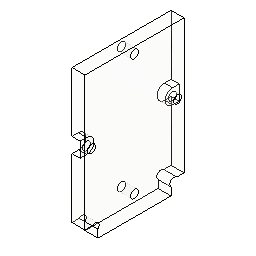
AssemblyThrowerNew v12 (Autodesk Fusion 360 archive; units mm, degrees)
design "RampBack"
Autodesk Fusion 360 part; units mm, degrees
sketch "Sketch1" plane through (0, 0, 0) normal (1, 0, 0) x (0, 1, 0)
  line L0 (-18.3, 27.3) -> (18.3, 27.3)
  line L1 (18.3, 27.3) -> (18.3, -22.3)
  line L2 (13.5, -27.3) -> (-13.5, -27.3)
  line L3 (-18.3, -22.3) -> (-18.3, 27.3)
  line L4 (0, 0) -> (0, 27.3) construction
  line L5 (-13.5, 27.3) -> (-13.5, -22.3) construction
  line L6 (13.5, 27.3) -> (13.5, -22.3) construction
  line L7 (-18.3, 22.5) -> (18.3, 22.5) construction
  line L8 (-18.3, -17.5) -> (18.3, -17.5) construction
  line L9 (-13.5, -22.3) -> (13.5, -22.3) construction
  line L10 (-18.3, 2.5) -> (18.3, 2.5) construction
  line L11 (0, 0) -> (0, -19.9) construction
  circle A0 centre (0, -19.9) radius 1.5
  circle A1 centre (-15.9, 2.5) radius 1.5
  circle A2 centre (15.9, 2.5) radius 1.5
  circle A3 centre (0, 24.9) radius 1.5
  line L12 (-18.3, -22.3) -> (-15.6213, -22.3)
  line L13 (-13.5, -24.4213) -> (-13.5, -27.3)
  line L14 (13.5, -24.4213) -> (13.5, -27.3)
  line L15 (15.6213, -22.3) -> (18.3, -22.3)
  line L16 (-18.3, -27.3) -> (-18.3, -22.3) construction
  line L17 (-13.5, -27.3) -> (-18.3, -27.3) construction
  line L18 (18.3, -27.3) -> (13.5, -27.3) construction
  line L19 (0, 0) -> (18.3, 0)
  line L20 (18.3, -22.3) -> (18.3, -27.3) construction
  line L21 (-13.5, -22.3) -> (-14.5607, -23.3607) construction
  arc A4 (-13.5, -24.4213) -> (-15.6213, -22.3) centre (-14.5607, -23.3607) ccw
  arc A5 (-15.6213, -22.3) -> (-13.5, -24.4213) centre (-14.5607, -23.3607) ccw construction
  line L22 (-13.5, -22.3) -> (-13.5, -24.4213) construction
  line L23 (-15.6213, -22.3) -> (-13.5, -22.3) construction
  line L24 (13.5, -22.3) -> (14.5607, -23.3607) construction
  arc A6 (15.6213, -22.3) -> (13.5, -24.4213) centre (14.5607, -23.3607) ccw
  arc A7 (13.5, -24.4213) -> (15.6213, -22.3) centre (14.5607, -23.3607) ccw construction
  line L25 (13.5, -22.3) -> (15.6213, -22.3) construction
  line L26 (13.5, -22.3) -> (13.5, -24.4213) construction
  line L27 (-15.9, -0.25) -> (-18.3, -0.25)
  line L28 (-15.9, 5.25) -> (-18.3, 5.25)
  arc A8 (-15.9, -0.25) -> (-15.9, 5.25) centre (-15.9, 2.5) ccw
  arc A9 (-15.9, 5.25) -> (-18.3, 3.8426) centre (-15.9, 2.5) ccw construction
  arc A10 (-18.3, 3.8426) -> (-18.3, 1.1574) centre (-15.9, 2.5) ccw construction
  arc A11 (-18.3, 1.1574) -> (-15.9, -0.25) centre (-15.9, 2.5) ccw construction
  line L29 (15.9, 5.25) -> (18.3, 5.25)
  line L30 (15.9, -0.25) -> (18.3, -0.25)
  arc A12 (15.9, -0.25) -> (15.9, 5.25) centre (15.9, 2.5) ccw construction
  arc A13 (14.7544, 0) -> (15.9, -0.25) centre (15.9, 2.5) ccw
  arc A14 (13.5, 1.1574) -> (14.7544, 0) centre (15.9, 2.5) ccw
  arc A15 (13.15, 2.5) -> (13.5, 1.1574) centre (15.9, 2.5) ccw
  arc A16 (13.5, 3.8426) -> (13.15, 2.5) centre (15.9, 2.5) ccw
  arc A17 (15.9, 5.25) -> (13.5, 3.8426) centre (15.9, 2.5) ccw
  point P0 (18.3, 0)
  dimension "d20" = 4.8
  dimension "d21" = 4.8
  dimension "d22" = 4.8
  dimension "d23" = 27
  dimension "d24" = 4.8
  dimension "d25" = 5
  dimension "d26" = 40
  dimension "d27" = 20
  dimension "d28" = 2.4
  dimension "d29" = 3
  dimension "d30" = 3
  dimension "d31" = 3
  dimension "d32" = 3
  dimension "d33" = 2.4
  dimension "d34" = 2.4
  dimension "d35" = 2.4
  dimension "d38" = 2.5
  dimension "d39" = 1.5
  dimension "d40" = 45
  dimension "d41" = 3
  dimension "d42" = 1.5
  dimension "d43" = 45
  dimension "d44" = 3
  dimension "d45" = 5.5
  dimension "d46" = 5.5
  constraint horizontal L0
  constraint vertical L1
  constraint horizontal L2
  constraint vertical L3
  constraint coincident L4.start L11.start
  constraint midpoint L0 L4.end
  constraint vertical L4
  constraint coincident L0 L5.start
  constraint perpendicular L2 L5
  constraint coincident L0 L6.start
  constraint perpendicular L2 L6
  constraint coincident L3 L7.start
  constraint coincident L1 L7.end
  constraint perpendicular L1 L7
  constraint coincident L3 L8.start
  constraint coincident L1 L8.end
  constraint perpendicular L1 L8
  constraint perpendicular L1 L9
  constraint coincident L3 L10.start
  constraint coincident L1 L10.end
  constraint perpendicular L1 L10
  constraint perpendicular L8 L11
  constraint coincident L11.end A0.centre
  constraint coincident L10 A1.centre
  constraint coincident L10 A2.centre
  constraint coincident L4 A3.centre
  constraint perpendicular L1 L12
  constraint perpendicular L2 L13
  constraint perpendicular L2 L14
  constraint perpendicular L1 L15
  constraint vertical L16
  constraint horizontal L17
  constraint horizontal L18
  constraint coincident L1 P0
  constraint coincident P0 L19.end
  constraint perpendicular L1 L19
  constraint vertical L20
  constraint coincident L21.end A4.centre
  constraint concentric A4 A5
  constraint perpendicular L2 L22
  constraint perpendicular L1 L23
  constraint coincident L24.end A6.centre
  constraint concentric A6 A7
  constraint perpendicular L1 L25
  constraint perpendicular L2 L26
  constraint concentric A1 A8
  constraint coincident L3 L27.end
  constraint tangent L27 A8
  constraint horizontal L27
  constraint coincident L3 L28.end
  constraint perpendicular L3 L28
  constraint tangent L28 A8
  constraint coincident L3 A9.end
  constraint concentric A8 A9
  constraint coincident L3 A10.end
  constraint concentric A8 A10
  constraint concentric A8 A11
  constraint concentric A2 A12
  constraint coincident L1 L29.end
  constraint perpendicular L1 L29
  constraint tangent L29 A12
  constraint coincident L1 L30.end
  constraint horizontal L30
  constraint tangent L30 A12
  constraint coincident L19 A13.start
  constraint concentric A12 A13
  constraint coincident L6 A14.start
  constraint concentric A12 A14
  constraint coincident L10 A15.start
  constraint concentric A12 A15
  constraint coincident L6 A16.start
  constraint concentric A12 A16
  constraint concentric A12 A17
  measures "d20" distance of L3 L5
  measures "d21" distance of L1 L6
  measures "d22" distance of L0 L7
  measures "d23" distance of L5 L6
  measures "d24" distance of L8 L9
  measures "d25" distance of L2 L9
  measures "d26" distance of L7 L8
  measures "d27" distance of L7 L10
  measures "d28" distance of L8 L11.end
  measures "d29" diameter of A0
  measures "d30" diameter of A1
  measures "d31" diameter of A2
  measures "d32" diameter of A3
  measures "d33" distance of L0 A3.centre
  measures "d34" distance of L3 A1.centre
  measures "d35" distance of L1 A2.centre
  measures "d38" distance of L10 P0
  measures "d39" distance of L5.end L21.end
  measures "d40" angle of L12 L21
  measures "d41" diameter of A4
  measures "d42" distance of L6.end L24.end
  measures "d43" angle of L15 L24
  measures "d44" diameter of A6
  measures "d45" diameter of A8
  measures "d46" diameter of A12
extrude "Extrude1" add sketch "Sketch1" along normal blind 4.8
extrude "Extrude2" cut sketch "Sketch1" along normal blind 3 contours L3 L27 L28 A8 | L1 L19 L29 A14 A15 A16 A17 | L1 L19 L30 A13

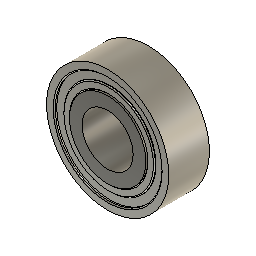
design "RollerBearing12x5x4"
Autodesk Fusion 360 part; units mm, degrees
sketch "Sketch1" plane through (0, 0, 0) normal (0, 1, 0) x (1, 0, 0)
  circle A0 centre (0, 0) radius 2.5
  circle A1 centre (0, 0) radius 3.75
  circle A2 centre (0, 0) radius 6
  circle A3 centre (0, 0) radius 5.25
  circle A4 centre (0, 0) radius 4.5
  dimension "d1" = 5
  dimension "d2" = 7.5
  dimension "d3" = 12
  dimension "d4" = 10.5
  dimension "d13" = 9
  constraint coincident A0.centre A1.centre
  constraint concentric A1 A2
  constraint concentric A1 A3
  constraint concentric A2 A4
  measures "d1" diameter of A0
  measures "d2" diameter of A1
  measures "d3" diameter of A2
  measures "d4" diameter of A3
  measures "d13" diameter of A4
extrude "Extrude1" add sketch "Sketch1" along normal blind 4 contours A2 | A3 | A4 makes body 1
extrude "Extrude2" add sketch "Sketch1" along normal blind 4 separate body contours A1 makes body 2
extrude "Extrude3" cut sketch "Sketch1" along normal blind 0.25 contours A3 bodies 1
sketch "Sketch2" plane through (0, 4, 0) normal (0, 1, 0) x (-1, 0, 0)
  circle A0 centre (0, 0) radius 3.75
  circle A1 centre (0, 0) radius 6
  circle A2 centre (0, 0) radius 5.25
  circle A3 centre (0, 0) radius 4.5
extrude "Extrude4" cut sketch "Sketch2" against normal blind 0.25 contours A2 bodies 1
extrude "Extrude5" cut 1 faces at (4.2193, 0, 0.4099) along direction (0, 1, 0) blind 0.1 on bodies 1 bodies 1
extrude "Extrude6" cut 1 faces at (-4.2193, 4, -0.4099) along direction (0, -1, 0) blind 0.1 on bodies 1 bodies 1
fillet "Fillet2" radius 0.1 6 edges at (-3.4962, 3.9, 1.3561) (4.1955, 3.9, 1.6273) (4.8947, 4, 1.8985) (-4.8947, 0, 1.8985) (-4.1955, 0.1, 1.6273) (-3.4962, 0.1, -1.3561) on bodies 1

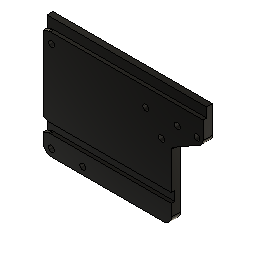
design "ThrowerStatorSidePlate"
Autodesk Fusion 360 part; units mm, degrees
sketch "Sketch1" plane through (0, 0, 0) normal (0, 1, 0) x (1, 0, 0)
  circle A0 centre (0, 0) radius 48 construction
  circle A1 centre (0, 0) radius 14 construction
  circle A2 centre (0, 0) radius 9.5 construction
  circle A3 centre (0, 0) radius 8 construction
  line L0 (0, 0) -> (8, 0) construction
  line L1 (0, 0) -> (0, -9.5) construction
  line L2 (0, 0) -> (-8, 0) construction
  line L3 (0, 0) -> (0, 9.5) construction
  circle A4 centre (8, 0) radius 1.5
  circle A5 centre (-8, 0) radius 1.5
  circle A6 centre (0, 9.5) radius 1.5
  circle A7 centre (0, 0) radius 12 construction
  line L4 (8, 0) -> (18, 0) construction
  line L5 (21.1, 0) -> (19.55, 2.6847) construction
  line L6 (19.55, 2.6847) -> (16.45, 2.6847) construction
  line L7 (16.45, 2.6847) -> (14.9, 0) construction
  line L8 (14.9, 0) -> (16.45, -2.6847) construction
  line L9 (16.45, -2.6847) -> (19.55, -2.6847) construction
  line L10 (19.55, -2.6847) -> (21.1, 0) construction
  circle A8 centre (18, 0) radius 3.1 construction
  circle A9 centre (18, 0) radius 1.5
  line L11 (0, 52) -> (-68, 52) construction
  line L12 (-9.7468, 47) -> (-68, 47) construction
  line L13 (-68, 52) -> (-68, 47) construction
  line L14 (-68, 47) -> (-68, 35.633) construction
  line L15 (-68, 35.633) -> (-32.1604, 35.633) construction
  line L16 (-68, 35.633) -> (-68, 30.833) construction
  line L17 (-68, 30.833) -> (-36.7876, 30.833) construction
  line L18 (-68, 30.833) -> (-68, -9.167) construction
  line L19 (-60, -9.167) -> (-47.1165, -9.167)
  line L20 (-68, -9.167) -> (-68, -13.967) construction
  line L21 (-68, -13.967) -> (-45.923, -13.967) construction
  line L22 (-60, -13.967) -> (-60, 35.633)
  line L23 (5.9333, 10.4305) -> (19.5328, 2.6945)
  line L24 (-60, -13.967) -> (21.1, -13.967)
  line L25 (21.1, -13.967) -> (21.1, 0)
  arc A10 (21.1, 0) -> (19.5328, 2.6945) centre (18, 0) ccw
  line L26 (-57, 35.633) -> (5, 35.633)
  line L27 (5, 35.633) -> (5, 11.8322)
  arc A11 (5.9333, 10.4305) -> (5.7778, 10.5175) centre (0, 0) ccw
  arc A12 (5, 11.8322) -> (5.7778, 10.5175) centre (6.5, 11.8322) ccw
  arc A13 (5.7778, 10.5175) -> (7.9656, 11.513) centre (6.5, 11.8322) ccw construction
  arc A14 (5.4445, 12.898) -> (5, 11.8322) centre (6.5, 11.8322) ccw construction
  arc A15 (7.9656, 11.513) -> (5.4445, 12.898) centre (6.5, 11.8322) ccw construction
  line L28 (5, 11.8322) -> (5, 10.9087) construction
  arc A16 (5.7778, 10.5175) -> (5, 10.9087) centre (0, 0) ccw construction
  line L29 (-57, 30.833) -> (5, 30.833)
  line L30 (-47.1165, -9.167) -> (21.1, -9.167)
  line L31 (-60, 35.633) -> (-60, 45.633)
  line L32 (-60, 45.633) -> (5, 45.633)
  line L33 (5, 45.633) -> (5, 35.633)
  circle A17 centre (-56, 42) radius 1.5
  circle A18 centre (-40, 42) radius 1.5
  line L34 (-40, 42) -> (0, 0) construction
  circle A19 centre (-55.8448, -4.167) radius 1.5
  line L35 (0, 0) -> (-55.8448, -4.167) construction
  line L36 (-68, -9.167) -> (-60, -9.167) construction
  line L37 (-57, -9.167) -> (-60, -8.167)
  line L38 (-57, -9.167) -> (-57, 30.833) construction
  line L39 (-57, 30.833) -> (-57, 35.633) construction
  line L40 (-57, 30.833) -> (-60, 29.833)
  line L41 (-57, 35.633) -> (-60, 36.633)
  line L42 (-60, 35.633) -> (-57, 35.633) construction
  line L43 (-60, 30.833) -> (-57, 30.833) construction
  point P0 (18, 0)
  point P1 (-33.1034, 34.7586)
  point P2 (-47.8669, -3.5717)
  dimension "d1" = 96
  dimension "d2" = 28
  dimension "d3" = 19
  dimension "d4" = 16
  dimension "d5" = 3
  dimension "d6" = 3
  dimension "d7" = 3
  dimension "d8" = 24
  dimension "d9" = 18
  dimension "d10" = 3.1
  dimension "d11" = 60
  dimension "d12" = 3
  dimension "d13" = 52
  dimension "d14" = 68
  dimension "d15" = 68
  dimension "d18" = 5
  dimension "d22" = 16.367
  dimension "d23" = 4.8
  dimension "d24" = 40
  dimension "d25" = 4.8
  dimension "d26" = 8
  dimension "d27" = 3.1
  dimension "d28" = 5
  dimension "d33" = 12
  dimension "d34" = 3
  dimension "d35" = 10
  dimension "d36" = 3
  dimension "d37" = 12
  dimension "d38" = 5
  dimension "d39" = 3
  dimension "d40" = 5
  dimension "d41" = 10
  dimension "d42" = 3
  dimension "d43" = 5
  dimension "d44" = 8
  dimension "d54" = 1
  dimension "d55" = 3
  dimension "d56" = 1
  dimension "d57" = 1
  constraint coincident A0.centre A1.centre
  constraint concentric A1 A3
  constraint coincident A3 L0.end
  constraint horizontal L0
  constraint coincident A2 L1.end
  constraint perpendicular L0 L1
  constraint coincident A3 L2.end
  constraint perpendicular L1 L2
  constraint coincident A2 L3.end
  constraint perpendicular L2 L3
  constraint coincident L0.end A4.centre
  constraint coincident L2.end A5.centre
  constraint coincident L3.end A6.centre
  constraint concentric A2 A7
  constraint parallel L0 L4
  constraint coincident P0 L4.end
  constraint coincident L8.end A8
  constraint horizontal L11
  constraint coincident A0 L12.start
  constraint parallel L11 L12
  constraint perpendicular L12 L13
  constraint perpendicular L12 L14
  constraint coincident A0 L15.end
  constraint perpendicular L14 L15
  constraint perpendicular L15 L16
  constraint coincident A0 L17.end
  constraint perpendicular L16 L17
  constraint perpendicular L17 L18
  constraint coincident A0 L19.end
  constraint perpendicular L18 L19
  constraint perpendicular L19 L20
  constraint coincident A0 L21.end
  constraint perpendicular L20 L21
  constraint coincident L21 L22.start
  constraint coincident L15 L22.end
  constraint perpendicular L15 L22
  constraint coincident A7 L23.start
  constraint coincident A8 L23.end
  constraint tangent A8 L23
  constraint tangent A7 L23
  constraint perpendicular L22 L24
  constraint tangent A8 L25
  constraint perpendicular L22 L26
  constraint coincident A7 L28.end
  constraint vertical L27
  constraint tangent L27 A13
  constraint tangent A11 A13
  constraint coincident A7 A11.end
  constraint concentric A12 A13
  constraint coincident A1 A13.end
  constraint coincident A1 A14.start
  constraint concentric A13 A14
  constraint concentric A13 A15
  constraint vertical L28
  constraint concentric A11 A16
  constraint coincident L27 L29.end
  constraint perpendicular L27 L29
  constraint coincident L25 L30.end
  constraint perpendicular L25 L30
  constraint perpendicular L15 L31
  constraint perpendicular L27 L32
  constraint perpendicular L26 L33
  constraint coincident A18.centre L34.start
  constraint coincident A0 P1
  constraint coincident L34 P1
  constraint coincident A19.centre L35.end
  constraint coincident L35 P2
  constraint coincident A0 P2
  constraint coincident L22 L19.start
  constraint perpendicular L18 L36
  constraint coincident L22 L43.start
  constraint coincident L17.end L29
  constraint coincident L19 L37.start
  constraint coincident L22 L37.end
  constraint coincident L17 L29.start
  constraint coincident L15 L26.start
  constraint coincident L22 L40.end
  constraint coincident L31 L41.end
  constraint vertical L38
  constraint vertical L39
  measures "d1" diameter of A0
  measures "d2" diameter of A1
  measures "d3" diameter of A2
  measures "d4" diameter of A3
  measures "d5" diameter of A4
  measures "d6" diameter of A5
  measures "d7" diameter of A6
  measures "d8" diameter of A7
  measures "d9" distance of A0.centre P0
  measures "d10" distance of L5.start P0
  measures "d11" angle of L4 L8
  measures "d12" diameter of A9
  measures "d13" distance of A0.centre L11
  measures "d14" horizontal distance of A0.centre L11.end
  measures "d15" distance of L11.start L11.end
  measures "d18" distance of L11 L12
  measures "d22" distance of L11 L15
  measures "d23" distance of L14.end L16.end
  measures "d24" distance of L16.end L18.end
  measures "d25" distance of L18.end L20.end
  measures "d26" distance of L18 L22
  measures "d27" radius of A10
  measures "d28" horizontal distance of A0.centre L26.end
  measures "d33" radius of A11
  measures "d34" diameter of A13
  measures "d35" distance of L15 L32
  measures "d36" diameter of A17
  measures "d37" distance of L14 A17.centre
  measures "d38" distance of L12 A17.centre
  measures "d39" diameter of A18
  measures "d40" distance of L12 A18.centre
  measures "d41" distance of A18.centre P1
  measures "d42" diameter of A19
  measures "d43" distance of L19 A19.centre
  measures "d44" distance of A19.centre P2
  measures "d54" distance of L19.start L37.end L3
  measures "d55" distance of L31 L26.start
  measures "d56" distance of L22.end L41.end L3
  measures "d57" distance of L43.start L40.end L3
extrude "Extrude1" add sketch "Sketch1" along normal blind 4.8
fillet "Fillet1" radius 4 2 edges at (5, 2.4, -45.633) (-60, 2.4, -45.633)
extrude "Extrude2" cut sketch "Sketch1" along normal blind 1.8 contours L19 L22 L37 | L19 L22 L24 L25 L30 | L22 L26 L27 L29 L31 L40 L41
fillet "Fillet2" radius 3 3 edges at (-57, 0.9, -35.633) (-57, 0.9, -30.833) (-57, 0.9, 9.167)

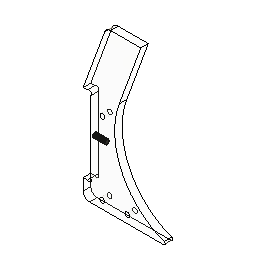
design "RampNew"
Autodesk Fusion 360 part; units mm, degrees
sketch "Sketch1" plane through (0, 0, 0) normal (0, 1, 0) x (1, 0, 0)
  line L0 (0, 0) -> (-48, 0) construction
  line L1 (-48, 0) -> (-68, 0) construction
  line L2 (0, 0) -> (0, 52) construction
  line L3 (-9.7468, 47) -> (-68, 47)
  line L4 (-68, 47) -> (-68, 0) construction
  line L5 (-45.1052, -16.417) -> (-31.4244, -54.0047)
  line L6 (-53.4275, -54.0047) -> (-68, -54.0047) construction
  line L7 (-68, -54.0047) -> (-68, 0) construction
  line L8 (-53.4275, -54.0047) -> (-68, -13.967)
  line L9 (-100, 35.633) -> (-100, 30.833) construction
  line L10 (-100, 30.833) -> (0, 30.833) construction
  line L11 (0, 0) -> (0, -9.167) construction
  line L12 (0, -9.167) -> (-100, -9.167) construction
  line L13 (-100, -9.167) -> (-100, -13.967) construction
  line L14 (0, -13.967) -> (0, -9.167) construction
  line L15 (-100, -9.167) -> (-100, 30.833) construction
  arc A0 (-9.7468, 47) -> (-45.1052, -16.417) centre (0, 0) ccw
  arc A1 (-45.1052, -16.417) -> (0, 48) centre (0, 0) ccw construction
  arc A2 (0, 48) -> (-9.7468, 47) centre (0, 0) ccw construction
  line L16 (-31.4244, -54.0047) -> (-53.4275, -54.0047)
  line L17 (-63.2, 35.633) -> (-63.2, -13.967)
  line L18 (0, 35.633) -> (-63.2, 35.633) construction
  line L19 (-68, 35.633) -> (-100, 35.633) construction
  line L20 (-65.3213, 35.633) -> (-68, 35.633)
  line L21 (-68, 47) -> (-68, 35.633)
  line L22 (-100, -13.967) -> (-68, -13.967) construction
  line L23 (-63.2, -13.967) -> (0, -13.967) construction
  line L24 (-68, -13.967) -> (-65.3213, -13.967)
  line L25 (0, 0) -> (-40, 42) construction
  line L26 (-40, 42) -> (-40, 47) construction
  circle A3 centre (-40, 42) radius 1.5
  circle A4 centre (-56, 42) radius 1.5
  line L27 (0, 0) -> (-55.8448, -4.167) construction
  line L28 (-55.8448, -4.167) -> (-55.8448, -9.167) construction
  circle A5 centre (-55.8448, -4.167) radius 1.5
  line L29 (-100, 10.833) -> (-63.2, 10.833) construction
  line L30 (-63.2, 10.833) -> (-55.2, 10.833) construction
  line L31 (-55.2, 9.333) -> (-55.2, 12.333) construction
  line L32 (-64.2607, -12.9063) -> (-63.2, -13.967) construction
  arc A6 (-65.3213, -13.967) -> (-63.2, -11.8457) centre (-64.2607, -12.9063) ccw
  arc A7 (-63.2, -11.8457) -> (-65.3213, -13.967) centre (-64.2607, -12.9063) ccw construction
  line L33 (-65.3213, -13.967) -> (-63.2, -13.967) construction
  line L34 (-63.2, 35.633) -> (-64.2607, 34.5723) construction
  arc A8 (-63.2, 33.5117) -> (-65.3213, 35.633) centre (-64.2607, 34.5723) ccw
  arc A9 (-65.3213, 35.633) -> (-63.2, 33.5117) centre (-64.2607, 34.5723) ccw construction
  line L35 (-63.2, 35.633) -> (-65.3213, 35.633) construction
  point P0 (-68, -13.967)
  point P1 (-33.1034, 34.7586)
  point P2 (-47.8669, -3.5717)
  point P3 (-100, 10.833)
  point P4 (-55.2, 10.833)
  dimension "d1" = 96
  dimension "d2" = 20
  dimension "d3" = 52
  dimension "d4" = 5
  dimension "d5" = 40
  dimension "d6" = 70
  dimension "d8" = 4.8
  dimension "d9" = 16.367
  dimension "d10" = 100
  dimension "d11" = 4.8
  dimension "d12" = 40
  dimension "d14" = 4.8
  dimension "d15" = 5
  dimension "d16" = 10
  dimension "d17" = 3
  dimension "d18" = 3
  dimension "d19" = 12
  dimension "d20" = 5
  dimension "d21" = 8
  dimension "d22" = 5
  dimension "d23" = 3
  dimension "d24" = 8
  dimension "d25" = 3
  dimension "d43" = 3
  dimension "d44" = 1.5
  dimension "d45" = 45
  dimension "d46" = 1.5
  dimension "d47" = 45
  constraint coincident L0.start L2.start
  constraint coincident L0.end A0
  constraint horizontal L0
  constraint parallel L0 L1
  constraint perpendicular L0 L2
  constraint parallel L1 L3
  constraint perpendicular L1 L4
  constraint tangent L5 A0
  constraint perpendicular L4 L6
  constraint perpendicular L1 L7
  constraint coincident L7 P0
  constraint parallel L5 L8
  constraint coincident L2 L18.start
  constraint perpendicular L2 L18
  constraint perpendicular L9 L18
  constraint coincident L2 L10.end
  constraint perpendicular L2 L10
  constraint perpendicular L0 L11
  constraint perpendicular L9 L12
  constraint perpendicular L12 L13
  constraint perpendicular L13 L22
  constraint perpendicular L12 L14
  constraint perpendicular L10 L15
  constraint coincident P0 L22
  constraint coincident L8 P0
  constraint coincident L2 A1.end
  constraint concentric A0 A1
  constraint concentric A0 A2
  constraint perpendicular L4 L16
  constraint coincident L17.start L18.end
  constraint coincident L17.end L22
  constraint perpendicular L17 L22
  constraint coincident L4 L19.start
  constraint parallel L10 L19
  constraint collinear L18 L20
  constraint collinear L23 L24
  constraint coincident L3 L26.end
  constraint perpendicular L3 L26
  constraint coincident L25 P1
  constraint coincident A0 P1
  constraint coincident L25.end L26.start
  constraint coincident L12 L28.end
  constraint perpendicular L12 L28
  constraint coincident A0 P2
  constraint coincident L27 P2
  constraint coincident L27.end L28.start
  constraint midpoint L15 P3
  constraint coincident P3 L29.start
  constraint midpoint L17 L29.end
  constraint perpendicular L17 L30
  constraint perpendicular L30 L31
  constraint midpoint L31 P4
  constraint coincident P4 L30.end
  constraint coincident L32.start A6.centre
  constraint coincident L17 A6.end
  constraint concentric A6 A7
  constraint collinear L23 L33
  constraint coincident L34.end A8.centre
  constraint coincident L17.start A8
  constraint coincident L17 A8.start
  constraint concentric A8 A9
  constraint collinear L18 L35
  measures "d1" diameter of A0
  measures "d2" distance of L0.end L1.end
  measures "d3" distance of L0.start L2.end
  measures "d4" distance of L2.end L3
  measures "d5" distance of L5.start L5.end
  measures "d6" angle of L0 L5
  measures "d8" distance of L9.start L9.end
  measures "d9" distance of L2.end L18
  measures "d10" distance of L18.start L9.start
  measures "d11" distance of L12.end L13.end
  measures "d12" distance of L9.end L12.end
  measures "d14" distance of L4 L17.start
  measures "d15" distance of L25.end L26.end
  measures "d16" distance of L25.end P1
  measures "d17" diameter of A3
  measures "d18" diameter of A4
  measures "d19" distance of L4 A4.centre
  measures "d20" distance of L3 A4.centre
  measures "d21" distance of L27.end P2
  measures "d22" distance of L27.end L28.end
  measures "d23" diameter of A5
  measures "d24" distance of L29.end P4
  measures "d25" distance of L31.start L31.end
  measures "d43" diameter of A6
  measures "d44" distance of L17.end L32.start
  measures "d45" angle of L24 L32
  measures "d46" distance of L17.start L34.end
  measures "d47" angle of L20 L34
extrude "Extrude1" add sketch "Sketch1" along normal blind 4.8 contours L3 L5 L8 A0 L16 L17 L20 L21 L24 A6 A8
sketch "Sketch2" plane through (-63.2, 0, 0) normal (-1, 0, 0) x (0, -1, 0)
  line L0 (0, -33.5117) -> (0, 11.8457)
  line L1 (-4.8, 11.8457) -> (-4.8, -33.5117)
  line L2 (0, -10.833) -> (-2.4, -10.833) construction
  circle A0 centre (-2.4, -10.833) radius 1.5
  line L3 (0, 11.8457) -> (-4.8, 11.8457)
  line L4 (-4.8, -33.5117) -> (0, -33.5117)
  point P0 (0, -10.833)
  dimension "d35" = 2.4
  dimension "d36" = 3
  constraint coincident P0 L2.start
  constraint perpendicular L0 L2
  constraint coincident L2.end A0.centre
  measures "d35" distance of P0 L2.end
  measures "d36" diameter of A0
extrude "Extrude2" cut sketch "Sketch2" against normal blind 8 contours A0
fillet "Fillet1" radius 4 1 edges at (-68, 2.4, -47)
fillet "Fillet1" radius 4 1 edges at (-53.4275, 2.4, 54.0047)
thread "Thread1" "ISO Metric profile 3.0 M3x0.5 6H" major diameter 3.086 minor diameter 2.529 pitch 0.5 angle 60 modelled right hand crest width 0.1368 on face at (-60.5333, 0.9075, -10.9824) crest through (-63.075, 1.1355, -10.833)
fillet "Fillet2" radius 1 1 edges at (-9.7468, 2.4, -47)

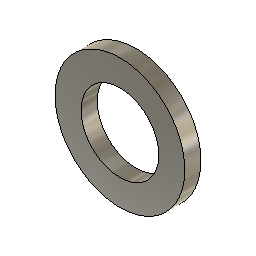
design "WasherM5"
Autodesk Fusion 360 part; units mm, degrees
sketch "Sketch1" plane through (0, 0, 0) normal (0, 1, 0) x (1, 0, 0)
  circle A0 centre (0, 0) radius 2.65
  circle A1 centre (0, 0) radius 4.425
  dimension "d1" = 5.3
  dimension "d2" = 8.85
  constraint coincident A0.centre A1.centre
  measures "d1" diameter of A0
  measures "d2" diameter of A1
extrude "Extrude1" add sketch "Sketch1" along normal blind 1.1

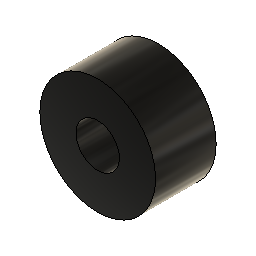
design "RampSpacer"
Autodesk Fusion 360 part; units mm, degrees
sketch "Sketch1" plane through (0, 0, 0) normal (0, 1, 0) x (1, 0, 0)
  circle A0 centre (0, 0) radius 1.5
  circle A1 centre (0, 0) radius 4
  dimension "d1" = 3
  dimension "d2" = 8
  constraint coincident A0.centre A1.centre
  constraint concentric A0 A1
  measures "d1" diameter of A0
  measures "d2" diameter of A1
extrude "Extrude1" add sketch "Sketch1" along normal blind 4.2

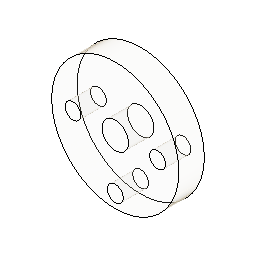
design "StatorSpacer"
Autodesk Fusion 360 part; units mm, degrees
sketch "Sketch1" plane through (0, 0, 0) normal (0, 1, 0) x (1, 0, 0)
  circle A0 centre (0, 0) radius 12
  circle A1 centre (0, 0) radius 9.5 construction
  circle A2 centre (0, 0) radius 8 construction
  line L0 (0, 0) -> (0, -9.5) construction
  line L1 (0, 0) -> (0, 9.5) construction
  line L2 (0, 0) -> (8, 0) construction
  line L3 (0, 0) -> (-8, 0) construction
  circle A3 centre (0, 9.5) radius 1.5
  circle A4 centre (8, 0) radius 1.5
  circle A5 centre (-8, 0) radius 1.5
  circle A6 centre (0, 0) radius 2.5
  dimension "d1" = 24
  dimension "d2" = 19
  dimension "d3" = 16
  dimension "d5" = 3
  dimension "d6" = 3
  dimension "d7" = 3
  dimension "d10" = 5
  constraint coincident A0.centre A1.centre
  constraint concentric A0 A1
  constraint coincident A1 L0.end
  constraint vertical L0
  constraint coincident A1 L1.end
  constraint parallel L0 L1
  constraint coincident A2 L2.end
  constraint perpendicular L0 L2
  constraint coincident A2 L3.end
  constraint perpendicular L0 L3
  constraint coincident L1.end A3.centre
  constraint coincident L2.end A4.centre
  constraint coincident L3.end A5.centre
  constraint concentric A0 A6
  measures "d1" diameter of A0
  measures "d2" diameter of A1
  measures "d3" diameter of A2
  measures "d5" diameter of A3
  measures "d6" diameter of A4
  measures "d7" diameter of A5
  measures "d10" diameter of A6
extrude "Extrude1" add sketch "Sketch1" along normal blind 4.8

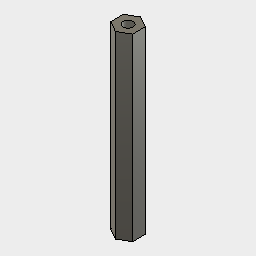
design "Spacer M3x45"
Autodesk Fusion 360 part; units mm, degrees
sketch "Sketch1" plane through (0, 0, 0) normal (0, 1, 0) x (1, 0, 0)
  line L0 (2.725, 1.5733) -> (0, 3.1466)
  line L1 (0, 3.1466) -> (-2.725, 1.5733)
  line L2 (-2.725, 1.5733) -> (-2.725, -1.5733)
  line L3 (-2.725, -1.5733) -> (0, -3.1466)
  line L4 (0, -3.1466) -> (2.725, -1.5733)
  line L5 (2.725, -1.5733) -> (2.725, 1.5733)
  circle A0 centre (0, 0) radius 1.25
  dimension "d1" = 2.5
  measures "d1" diameter of A0
extrude "Extrude1" add sketch "Sketch1" along normal blind 45

design "ThrowerRotorSidePlate"
Autodesk Fusion 360 part; units mm, degrees
sketch "Sketch1" plane through (0, 0, 0) normal (0, 1, 0) x (1, 0, 0)
  circle A0 centre (0, 0) radius 48 construction
  circle A1 centre (0, 0) radius 14 construction
  circle A2 centre (0, 0) radius 9.5 construction
  circle A3 centre (0, 0) radius 8 construction
  line L0 (0, 0) -> (8, 0) construction
  line L1 (0, 0) -> (0, -9.5) construction
  line L2 (0, 0) -> (-8, 0) construction
  line L3 (0, 0) -> (0, 9.5) construction
  circle A4 centre (8, 0) radius 1.5 construction
  circle A5 centre (-8, 0) radius 1.5 construction
  circle A6 centre (0, 9.5) radius 1.5 construction
  circle A7 centre (0, 0) radius 12 construction
  line L4 (8, 0) -> (18, 0) construction
  line L5 (21.1, 0) -> (19.55, 2.6847) construction
  line L6 (19.55, 2.6847) -> (16.45, 2.6847) construction
  line L7 (16.45, 2.6847) -> (14.9, 0) construction
  line L8 (14.9, 0) -> (16.45, -2.6847) construction
  line L9 (16.45, -2.6847) -> (19.55, -2.6847) construction
  line L10 (19.55, -2.6847) -> (21.1, 0) construction
  circle A8 centre (18, 0) radius 3.1 construction
  circle A9 centre (18, 0) radius 1.5
  line L11 (0, 52) -> (-68, 52) construction
  line L12 (-9.7468, 47) -> (-68, 47) construction
  line L13 (-68, 52) -> (-68, 47) construction
  line L14 (-68, 47) -> (-68, 35.633) construction
  line L15 (-68, 35.633) -> (-32.1604, 35.633) construction
  line L16 (-68, 35.633) -> (-68, 30.833) construction
  line L17 (-68, 30.833) -> (-36.7876, 30.833) construction
  line L18 (-68, 30.833) -> (-68, -9.167) construction
  line L19 (-60, -9.167) -> (-47.1165, -9.167)
  line L20 (-68, -9.167) -> (-68, -13.967) construction
  line L21 (-68, -13.967) -> (-45.923, -13.967) construction
  line L22 (-60, -13.967) -> (-60, 35.633)
  line L23 (5.9333, 10.4305) -> (19.5328, 2.6945)
  line L24 (-60, -13.967) -> (21.1, -13.967)
  line L25 (21.1, -13.967) -> (21.1, 0)
  arc A10 (21.1, 0) -> (19.5328, 2.6945) centre (18, 0) ccw
  line L26 (-60, 35.633) -> (5, 35.633)
  line L27 (5, 35.633) -> (5, 11.8322)
  arc A11 (5.9333, 10.4305) -> (5.7778, 10.5175) centre (0, 0) ccw
  arc A12 (5, 11.8322) -> (5.7778, 10.5175) centre (6.5, 11.8322) ccw
  arc A13 (5.7778, 10.5175) -> (7.9656, 11.513) centre (6.5, 11.8322) ccw construction
  arc A14 (5.4445, 12.898) -> (5, 11.8322) centre (6.5, 11.8322) ccw construction
  arc A15 (7.9656, 11.513) -> (5.4445, 12.898) centre (6.5, 11.8322) ccw construction
  line L28 (5, 11.8322) -> (5, 10.9087) construction
  arc A16 (5.7778, 10.5175) -> (5, 10.9087) centre (0, 0) ccw construction
  line L29 (-60, 30.833) -> (5, 30.833)
  line L30 (-47.1165, -9.167) -> (21.1, -9.167)
  line L31 (-60, 35.633) -> (-60, 45.633)
  line L32 (-60, 45.633) -> (5, 45.633)
  line L33 (5, 45.633) -> (5, 35.633)
  circle A17 centre (-56, 42) radius 1.5
  circle A18 centre (-40, 42) radius 1.5
  line L34 (-40, 42) -> (0, 0) construction
  circle A19 centre (-55.8448, -4.167) radius 1.5
  line L35 (0, 0) -> (-55.8448, -4.167) construction
  line L36 (-68, -9.167) -> (-60, -9.167) construction
  line L37 (-6, -7.5) -> (7.5, -7.5)
  line L38 (7.5, -7.5) -> (7.5, 7.5)
  line L39 (6, 7.5) -> (-7.5, 7.5)
  line L40 (-7.5, 7.5) -> (-7.5, -7.5)
  line L41 (-7.5, -7.5) -> (7.5, 7.5) construction
  line L42 (-7.5, 7.5) -> (7.5, -7.5) construction
  arc A20 (-7.5, -6) -> (-7.0607, -7.0607) centre (-6, -6) ccw
  arc A21 (-7.0607, -7.0607) -> (-6, -7.5) centre (-6, -6) ccw
  line L43 (-7.5, -7.5) -> (-6, -7.5)
  arc A22 (-6, -7.5) -> (-4.602, -6.5438) centre (-6, -6) ccw construction
  arc A23 (-4.9393, -4.9393) -> (-7.5, -6) centre (-6, -6) ccw construction
  arc A24 (-4.602, -6.5438) -> (-4.9393, -4.9393) centre (-6, -6) ccw construction
  arc A25 (6, -7.5) -> (7.0607, -7.0607) centre (6, -6) ccw
  arc A26 (7.0607, -7.0607) -> (7.5, -6) centre (6, -6) ccw
  arc A27 (7.5, -6) -> (6.5438, -4.602) centre (6, -6) ccw construction
  arc A28 (4.9393, -4.9393) -> (6, -7.5) centre (6, -6) ccw construction
  arc A29 (6.5438, -4.602) -> (4.9393, -4.9393) centre (6, -6) ccw construction
  arc A30 (7.0607, 7.0607) -> (6, 7.5) centre (6, 6) ccw
  arc A31 (7.5, 6) -> (7.0607, 7.0607) centre (6, 6) ccw
  arc A32 (6, 7.5) -> (6.5438, 4.602) centre (6, 6) ccw construction
  arc A33 (7.4916, 5.8417) -> (7.5, 6) centre (6, 6) ccw construction
  arc A34 (6.5438, 4.602) -> (7.4916, 5.8417) centre (6, 6) ccw construction
  arc A35 (-7.0607, 7.0607) -> (-7.5, 6) centre (-6, 6) ccw
  arc A36 (-6.8748, 7.2185) -> (-7.0607, 7.0607) centre (-6, 6) ccw
  arc A37 (-6, 7.5) -> (-6.8748, 7.2185) centre (-6, 6) ccw
  arc A38 (-7.5, 6) -> (-4.8256, 5.0669) centre (-6, 6) ccw construction
  arc A39 (-4.602, 6.5438) -> (-6, 7.5) centre (-6, 6) ccw construction
  arc A40 (-4.8256, 5.0669) -> (-4.602, 6.5438) centre (-6, 6) ccw construction
  line L44 (7.5, 7.5) -> (6, 7.5)
  point P0 (18, 0)
  point P1 (-33.1034, 34.7586)
  point P2 (-47.8669, -3.5717)
  dimension "d1" = 96
  dimension "d2" = 28
  dimension "d3" = 19
  dimension "d4" = 16
  dimension "d5" = 3
  dimension "d6" = 3
  dimension "d7" = 3
  dimension "d8" = 24
  dimension "d9" = 18
  dimension "d10" = 3.1
  dimension "d11" = 60
  dimension "d12" = 3
  dimension "d13" = 52
  dimension "d14" = 68
  dimension "d15" = 68
  dimension "d18" = 5
  dimension "d22" = 16.367
  dimension "d23" = 4.8
  dimension "d24" = 40
  dimension "d25" = 4.8
  dimension "d26" = 8
  dimension "d27" = 3.1
  dimension "d28" = 5
  dimension "d33" = 12
  dimension "d34" = 3
  dimension "d35" = 10
  dimension "d36" = 3
  dimension "d37" = 12
  dimension "d38" = 5
  dimension "d39" = 3
  dimension "d40" = 5
  dimension "d41" = 10
  dimension "d42" = 3
  dimension "d43" = 5
  dimension "d44" = 8
  dimension "d66" = 7.5
  dimension "d67" = 7.5
  dimension "d68" = 15
  dimension "d69" = 15
  dimension "d70" = 3
  dimension "d71" = 3
  dimension "d72" = 3
  dimension "d73" = 3
  constraint coincident A0.centre A1.centre
  constraint concentric A1 A3
  constraint coincident A3 L0.end
  constraint horizontal L0
  constraint coincident A2 L1.end
  constraint perpendicular L0 L1
  constraint coincident A3 L2.end
  constraint perpendicular L1 L2
  constraint coincident A2 L3.end
  constraint perpendicular L2 L3
  constraint coincident L0.end A4.centre
  constraint coincident L2.end A5.centre
  constraint coincident L3.end A6.centre
  constraint concentric A2 A7
  constraint parallel L0 L4
  constraint coincident P0 L4.end
  constraint coincident L8.end A8
  constraint horizontal L11
  constraint coincident A0 L12.start
  constraint parallel L11 L12
  constraint perpendicular L12 L13
  constraint perpendicular L12 L14
  constraint coincident A0 L15.end
  constraint perpendicular L14 L15
  constraint perpendicular L15 L16
  constraint coincident A0 L17.end
  constraint perpendicular L16 L17
  constraint perpendicular L17 L18
  constraint coincident A0 L19.end
  constraint perpendicular L18 L19
  constraint perpendicular L19 L20
  constraint coincident A0 L21.end
  constraint perpendicular L20 L21
  constraint coincident L21 L22.start
  constraint coincident L15 L22.end
  constraint perpendicular L15 L22
  constraint coincident A7 L23.start
  constraint coincident A8 L23.end
  constraint tangent A8 L23
  constraint tangent A7 L23
  constraint perpendicular L22 L24
  constraint tangent A8 L25
  constraint perpendicular L22 L26
  constraint coincident A7 L28.end
  constraint vertical L27
  constraint tangent L27 A13
  constraint tangent A11 A13
  constraint coincident A7 A11.end
  constraint concentric A12 A13
  constraint coincident A1 A13.end
  constraint coincident A1 A14.start
  constraint concentric A13 A14
  constraint concentric A13 A15
  constraint vertical L28
  constraint concentric A11 A16
  constraint coincident L27 L29.end
  constraint perpendicular L27 L29
  constraint coincident L25 L30.end
  constraint perpendicular L25 L30
  constraint perpendicular L15 L31
  constraint perpendicular L27 L32
  constraint perpendicular L26 L33
  constraint coincident A18.centre L34.start
  constraint coincident A0 P1
  constraint coincident L34 P1
  constraint coincident A19.centre L35.end
  constraint coincident L35 P2
  constraint coincident A0 P2
  constraint coincident L22 L19.start
  constraint perpendicular L18 L36
  constraint coincident L22 L29.start
  constraint coincident L17.end L29
  constraint horizontal L37
  constraint vertical L38
  constraint horizontal L39
  constraint vertical L40
  constraint coincident L41 A20.centre
  constraint tangent L37 A22
  constraint coincident L42 A25.centre
  constraint tangent L37 A27
  constraint coincident L41 A30.centre
  constraint tangent L39 A32
  constraint coincident L42 A35.centre
  constraint tangent L39 A38
  constraint coincident L40 A20.start
  constraint coincident L41 A20.end
  constraint concentric A20 A22
  constraint concentric A21 A22
  constraint horizontal L43
  constraint coincident A3 A22.end
  constraint coincident L41 A23.start
  constraint concentric A22 A23
  constraint concentric A22 A24
  constraint coincident L37 A25.start
  constraint coincident L42 A25.end
  constraint concentric A25 A27
  constraint coincident L38 A26.end
  constraint concentric A26 A27
  constraint coincident A3 A27.end
  constraint coincident L42 A28.start
  constraint concentric A27 A28
  constraint concentric A27 A29
  constraint coincident L41 A30.start
  constraint concentric A30 A32
  constraint coincident L38 A31.start
  constraint concentric A31 A32
  constraint coincident A3 A32.end
  constraint coincident A2 A33.start
  constraint concentric A32 A33
  constraint concentric A32 A34
  constraint coincident L42 A35.start
  constraint coincident L40 A35.end
  constraint concentric A35 A38
  constraint coincident L39 A37.start
  constraint coincident L34 A36.start
  constraint concentric A36 A38
  constraint concentric A37 A38
  constraint coincident L34 A38.end
  constraint coincident A3 A39.start
  constraint concentric A38 A39
  constraint concentric A38 A40
  constraint horizontal L44
  measures "d1" diameter of A0
  measures "d2" diameter of A1
  measures "d3" diameter of A2
  measures "d4" diameter of A3
  measures "d5" diameter of A4
  measures "d6" diameter of A5
  measures "d7" diameter of A6
  measures "d8" diameter of A7
  measures "d9" distance of A0.centre P0
  measures "d10" distance of L5.start P0
  measures "d11" angle of L4 L8
  measures "d12" diameter of A9
  measures "d13" distance of A0.centre L11
  measures "d14" horizontal distance of A0.centre L11.end
  measures "d15" distance of L11.start L11.end
  measures "d18" distance of L11 L12
  measures "d22" distance of L11 L15
  measures "d23" distance of L14.end L16.end
  measures "d24" distance of L16.end L18.end
  measures "d25" distance of L18.end L20.end
  measures "d26" distance of L18 L22
  measures "d27" radius of A10
  measures "d28" horizontal distance of A0.centre L26.end
  measures "d33" radius of A11
  measures "d34" diameter of A13
  measures "d35" distance of L15 L32
  measures "d36" diameter of A17
  measures "d37" distance of L14 A17.centre
  measures "d38" distance of L12 A17.centre
  measures "d39" diameter of A18
  measures "d40" distance of L12 A18.centre
  measures "d41" distance of A18.centre P1
  measures "d42" diameter of A19
  measures "d43" distance of L19 A19.centre
  measures "d44" distance of A19.centre P2
  measures "d66" distance of A0.centre L37
  measures "d67" distance of A0.centre L38
  measures "d68" distance of L40.end L37.end
  measures "d69" distance of L40.end L39.end
  measures "d70" diameter of A22
  measures "d71" diameter of A38
  measures "d72" diameter of A27
  measures "d73" diameter of A32
extrude "Extrude1" add sketch "Sketch1" along normal blind 4.8 contours L19 L22 L23 L25 A10 L27 A11 A12 L29 L30 | L19 L22 L24 L25 L30 | L22 L26 L27 L29 | L26 L31 L32 L33 | L40 A20 A21 L43 | L37 L38 A25 A26 | L39 L40 A35 A36 A37 | L38 A30 A31 L44
fillet "Fillet1" radius 4 2 edges at (5, 2.4, -45.633) (-60, 2.4, -45.633)
sketch "Sketch2" plane through (0, 4.8, 0) normal (0, 1, 0) x (-1, 0, 0)
  arc A0 (56, -45.633) -> (60, -41.633) centre (56, -41.633) ccw
  line L0 (60, -41.633) -> (60, 13.967)
  line L1 (60, 13.967) -> (-21.1, 13.967)
  line L2 (-21.1, 13.967) -> (-21.1, 0)
  arc A1 (-21.1, 0) -> (-19.5328, -2.6945) centre (-18, 0) ccw
  line L3 (-19.5328, -2.6945) -> (-5.9333, -10.4305)
  arc A2 (-5.9333, -10.4305) -> (-5.7778, -10.5175) centre (0, 0) ccw
  arc A3 (-5, -11.8322) -> (-5.7778, -10.5175) centre (-6.5, -11.8322) ccw
  line L4 (-5, -11.8322) -> (-5, -41.633)
  arc A4 (-5, -41.633) -> (-1, -45.633) centre (-1, -41.633) ccw
  line L5 (-1, -45.633) -> (56, -45.633)
  circle A5 centre (55.8448, 4.167) radius 1.5
  circle A6 centre (40, -42) radius 1.5
  circle A7 centre (56, -42) radius 1.5
  circle A8 centre (-18, 0) radius 1.5
  line L6 (47.1165, 9.167) -> (-21.1, 9.167)
  line L7 (60, 9.167) -> (47.1165, 9.167)
  line L8 (60, -30.833) -> (-5, -30.833)
  line L9 (60, -35.633) -> (-5, -35.633)
  line L10 (-21.1, 13.967) -> (60, 13.967)
  line L11 (60, 13.967) -> (60, 9.167)
  line L12 (57, 9.167) -> (-21.1, 9.167)
  line L13 (-21.1, 9.167) -> (-21.1, 13.967)
  line L14 (-5, -30.833) -> (57, -30.833)
  line L15 (60, -30.833) -> (60, -35.633)
  line L16 (57, -35.633) -> (-5, -35.633)
  line L17 (-5, -35.633) -> (-5, -30.833)
  line L18 (57, 9.167) -> (60, 8.167)
  line L19 (60, 8.167) -> (60, 9.167)
  line L20 (60, 9.167) -> (57, 9.167) construction
  line L21 (57, -30.833) -> (60, -29.833)
  line L22 (60, -30.833) -> (60, -29.833)
  line L23 (60, -35.633) -> (60, -36.633)
  line L24 (60, -36.633) -> (57, -35.633)
  line L25 (57, -35.633) -> (57, -30.833) construction
  line L26 (57, 9.167) -> (57, -30.833) construction
  line L27 (57, -30.833) -> (60, -30.833) construction
  line L28 (60, -35.633) -> (57, -35.633) construction
  arc A9 (6, -7.5) -> (7.5, -6) centre (6, -6) ccw
  line L29 (6, -7.5) -> (-6, -7.5)
  arc A10 (-7.5, -6) -> (-6, -7.5) centre (-6, -6) ccw
  line L30 (-7.5, -6) -> (-7.5, 6)
  arc A11 (-6, 7.5) -> (-7.5, 6) centre (-6, 6) ccw
  line L31 (-6, 7.5) -> (6, 7.5)
  arc A12 (7.5, 6) -> (6, 7.5) centre (6, 6) ccw
  line L32 (7.5, 6) -> (7.5, -6)
  dimension "d60" = 3
  dimension "d61" = 1
  dimension "d62" = 1
  dimension "d63" = 1
  constraint horizontal L10
  constraint vertical L11
  constraint horizontal L12
  constraint vertical L13
  constraint coincident L7.start L11.end
  constraint coincident L1.end L2.start
  constraint horizontal L14
  constraint vertical L15
  constraint horizontal L16
  constraint vertical L17
  constraint coincident L9.start L15.end
  constraint coincident L8.end L14.start
  constraint coincident L0 L18.end
  constraint horizontal L20
  constraint coincident L0 L21.end
  constraint coincident L0 L23.end
  constraint perpendicular L16 L23
  constraint vertical L26
  constraint vertical L25
  constraint horizontal L27
  constraint horizontal L28
  measures "d60" horizontal distance of L12.start L18.end
  measures "d61" distance of L7.start L18.end
  measures "d62" distance of L14 L21.end
  measures "d63" distance of L16 L23.end
extrude "Extrude4" cut sketch "Sketch2" against normal blind 1.8 contours L0 L9 L23 L24 | L0 L4 L8 L9 L14 L15 L16 L17 | L0 L8 L21 L22 | L0 L7 L18 L19 | L0 L1 L2 L6 L7 L10 L11 L12 L13
fillet "Fillet2" radius 3 3 edges at (-57, 3.9, 9.167) (-57, 3.9, -30.833) (-57, 3.9, -35.633)
